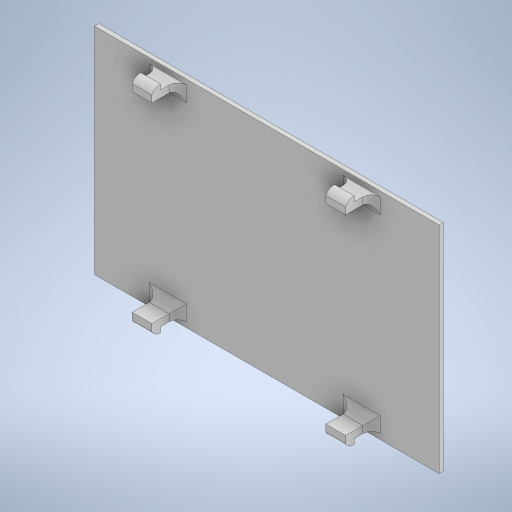
# Autodesk Inventor part: cover
Saved by Autodesk Inventor 2023 (Build 270158000, 158)
## iProperties
Created: 2022-11-06
Part Number: cover
Material: Generic
Document SubType Name: Modeling
Designer: omrfrkmll
Density: 1 g/cm^3
Appearance: Default
Author: omrfrkmll
Autodesk Inventor part; units mm, degrees
ref_plane "YZ Plane" through (0, 0, 0) normal (1, 0, 0) x (0, 1, 0)
ref_plane "XZ Plane" through (0, 0, 0) normal (0, 1, 0) x (-1, 0, 0)
sketch "Sketch1" plane through (0, 0, 0) normal (0, 0, 1) x (1, 0, 0)
  line L0 (0, 10.3664) -> (0, -9.7905)
  line L1 (-11.2303, 0) -> (9.7082, 0)
  line L2 (-40, 25) -> (40, 25)
  line L3 (40, 25) -> (40, -25)
  line L4 (40, -25) -> (-40, -25)
  line L5 (-40, -25) -> (-40, 25)
  point P0 (0, 0)
  dimension "d0" = 80
  dimension "d1" = 50
  constraints: 12 end point, 3 horizontal, 2 parallel, 2 vertical, 1 perpendicular, 2 other
  measures "d0" distance between parallel lines of L3 L5
  measures "d1" distance between parallel lines of L4 L2
extrude "Extrusion1" add sketch "Sketch1" along normal blind 1
sketch "Sketch2" plane through (0, 0, 1) normal (0, 0, 1) x (1, 0, 0)
  line L0 (-25.47, 29.9826) -> (-25.47, 14.8936)
  line L1 (-40, 25) -> (-40, -25) projected
  line L2 (-20.47, 29.2374) -> (-20.47, 19.4575)
  line L3 (19.53, 30.5414) -> (19.53, 15.3593)
  line L4 (40, -25) -> (40, 25) projected
  line L5 (24.53, 28.7717) -> (24.53, 17.8741)
  line L6 (-43.5467, 24) -> (46.149, 24)
  line L7 (40, 25) -> (-40, 25) projected
  line L8 (-25.47, 24) -> (-20.47, 24)
  line L9 (-20.47, 24) -> (-20.47, 22)
  line L10 (-20.47, 22) -> (-25.47, 22)
  line L11 (-25.47, 22) -> (-25.47, 24)
  line L12 (-25.27, 22.2) -> (-20.67, 22.2)
  line L13 (-20.67, 22.2) -> (-20.67, 23.8)
  line L14 (-20.67, 23.8) -> (-25.27, 23.8)
  line L15 (-25.27, 23.8) -> (-25.27, 22.2)
  line L16 (19.53, 24) -> (24.53, 24)
  line L17 (24.53, 24) -> (24.53, 22)
  line L18 (24.53, 22) -> (19.53, 22)
  line L19 (19.53, 22) -> (19.53, 24)
  line L20 (19.73, 22.2) -> (24.33, 22.2)
  line L21 (24.33, 22.2) -> (24.33, 23.8)
  line L22 (24.33, 23.8) -> (19.73, 23.8)
  line L23 (19.73, 23.8) -> (19.73, 22.2)
  point P0 (0, 0)
  dimension "d4" = 14.53
  dimension "d5" = 19.53
  dimension "d6" = 20.47
  dimension "d7" = 15.47
  dimension "d8" = 1
  dimension "d9" = 4
  dimension "d10" = 0.2
  dimension "d11" = 4
  dimension "d12" = 0.2
  constraints: 42 end point, 8 parallel, 6 point on line, 4 perpendicular, 4 vertical, 3 horizontal, 6 other
  measures "d4" distance between parallel lines of L1 L0
  measures "d5" distance between parallel lines of L1 L2
  measures "d6" distance between parallel lines of L4 L3
  measures "d7" distance between parallel lines of L4 L5
  measures "d8" distance between parallel lines of L7 L6
  measures "d9" diameter of L10 L6
  measures "d10" distance between parallel lines of L10 L12
  measures "d11" diameter of L18 L6
  measures "d12" distance between parallel lines of L18 L20
extrude "Extrusion2" add sketch "Sketch2" along normal blind 6 contours L15 L14 L13 L12 | L23 L22 L21 L20
sketch "Sketch4" plane through (-25.27, 22.2, 1) normal (-1, 0, 0) x (0, 0, 1)
  line L0 (0, 1.6) -> (6, 1.6) projected
  arc A0 (6, 1.6) -> (4, 2.8) centre (4.164, 0.8067) ccw
  line L1 (6, 1.6) -> (6, 0) projected
  line L2 (4, 2.8) -> (4, 1.6)
  line L3 (4, 1.6) -> (6, 1.6)
  point P0 (-1, -22.2)
  dimension "d15" = 1.2
  dimension "d16" = 2
  dimension "d17" = 2
  constraints: 4 end point, 2 perpendicular, 2 point on circle, 1 centre point, 1 point on line
  measures "d15" distance from line of L0 L2.start
  measures "d16" distance from line of L1 L2.start
  measures "d17" radius of A0
extrude "Extrusion3" add sketch "Sketch4" against normal up to surface (4.6 mm away)
ref_plane "Work Plane1" through (-0.47, 22.2, 1) normal (-1, 0, 0) x (0, 0, 1)
mirror "Mirror2" about plane through (0, 0, 0) normal (0, 1, 0) of "Extrusion3", "Extrusion2"
mirror "Mirror1" about plane through (-0.47, 22.2, 1) normal (-1, 0, 0) of "Extrusion3", "Extrusion2", "Mirror2"
fillet "Fillet1" radius 2 12 edges at (-20.67, -23, 1) (-22.97, -22.2, 1) (-25.27, -23, 1) (24.33, -23, 1) (22.03, -22.2, 1) (19.73, -23, 1) (19.73, 23, 1) (22.03, 22.2, 1) (24.33, 23, 1) (-20.67, 23, 1) (-22.97, 22.2, 1) (-25.27, 23, 1)
body "Solid1"
